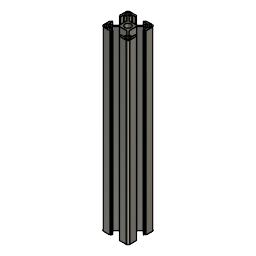
20cm profile beam (Autodesk Fusion 360 design; units mm, degrees)
Autodesk Fusion 360 part; units mm, degrees
sketch "Sketch1" plane through (0, 0, 0) normal (0, 0, 1) x (1, 0, 0)
  line L0 (-150, 300) -> (-150, 150) construction
  line L1 (0, 150) -> (-300, 150) construction
  line L2 (-205, 150) -> (-205, 192.65)
  line L3 (-191.8942, 205) -> (-108.1058, 205)
  line L4 (-95, 192.65) -> (-95, 150)
  line L5 (-150, 150) -> (-205, 205) construction
  line L6 (-150, 150) -> (-95, 205) construction
  line L7 (-205, 150) -> (-205, 192.65) construction
  line L8 (-280, 300) -> (-232.5, 300)
  line L9 (-232.5, 277) -> (-232.5, 246.4343)
  line L10 (-300, 232.5) -> (-300, 280)
  line L11 (-205, 192.65) -> (-244.2642, 231.9142)
  line L12 (-231.9142, 245.0201) -> (-191.8942, 205)
  line L13 (-279, 193) -> (-279, 232.5)
  line L14 (-288, 278) -> (-288, 150) construction
  line L15 (-278, 288) -> (-254.5, 288)
  line L16 (-244.5, 278) -> (-244.5, 254.5)
  line L17 (-254.5, 244.5) -> (-278, 244.5)
  arc A0 (-278, 288) -> (-288, 278) centre (-278, 278) ccw
  arc A1 (-244.5, 278) -> (-254.5, 288) centre (-254.5, 278) ccw
  arc A2 (-254.5, 244.5) -> (-244.5, 254.5) centre (-254.5, 254.5) ccw
  arc A3 (-288, 254.5) -> (-278, 244.5) centre (-278, 254.5) ccw
  line L18 (-288, 278) -> (-288, 254.5)
  line L19 (-191, 281) -> (-191, 286)
  line L20 (-200.9796, 290) -> (-200.9796, 298)
  line L21 (-193, 288) -> (-198.9796, 288)
  line L22 (-280, 300) -> (-202.9796, 300)
  line L23 (-230.5, 279) -> (-193, 279)
  line L24 (-279, 230.5) -> (-279, 191)
  line L25 (-288, 193) -> (-288, 198.6085)
  line L26 (-290, 200.6085) -> (-298, 200.6085)
  line L27 (-281, 191) -> (-286, 191)
  line L28 (-300, 280) -> (-300, 202.6085)
  line L29 (-288, 191) -> (-288, 288) construction
  line L30 (-245.6784, 232.5) -> (-277, 232.5)
  line L31 (-294.1421, 294.1421) -> (-285.0711, 285.0711) construction
  line L32 (-288, 288) -> (-285.0711, 285.0711) construction
  line L33 (-247.4289, 247.4289) -> (-150, 150) construction
  arc A4 (-200.9796, 298) -> (-202.9796, 300) centre (-202.9796, 298) ccw
  arc A5 (-191, 286) -> (-193, 288) centre (-193, 286) ccw
  arc A6 (-193, 279) -> (-191, 281) centre (-193, 281) ccw
  arc A7 (-200.9796, 290) -> (-198.9796, 288) centre (-198.9796, 290) ccw
  arc A8 (-230.5, 279) -> (-232.5, 277) centre (-230.5, 277) ccw
  arc A9 (-232.5, 246.4343) -> (-231.9142, 245.0201) centre (-230.5, 246.4343) ccw
  arc A10 (-244.2642, 231.9142) -> (-245.6784, 232.5) centre (-245.6784, 230.5) ccw
  line L34 (-300, 202.6085) -> (-300, 280)
  arc A11 (-288, 198.6085) -> (-290, 200.6085) centre (-290, 198.6085) ccw
  arc A12 (-288, 193) -> (-286, 191) centre (-286, 193) ccw
  arc A13 (-281, 191) -> (-279, 193) centre (-281, 193) ccw
  arc A14 (-277, 232.5) -> (-279, 230.5) centre (-277, 230.5) ccw
  arc A15 (-300, 202.6085) -> (-298, 200.6085) centre (-298, 202.6085) ccw
  arc A16 (-280, 300) -> (-300, 280) centre (-280, 280) ccw
  line L35 (-21, 193) -> (-21, 232.5)
  line L36 (-21, 230.5) -> (-21, 191)
  line L37 (-12, 191) -> (-12, 288) construction
  arc A17 (-12, 278) -> (-22, 288) centre (-22, 278) ccw
  line L38 (-68.0858, 245.0201) -> (-108.1058, 205)
  line L39 (0, 202.6085) -> (0, 280)
  arc A18 (-22, 244.5) -> (-12, 254.5) centre (-22, 254.5) ccw
  line L40 (-20, 300) -> (-97.0204, 300)
  line L41 (-95, 192.65) -> (-55.7358, 231.9142)
  arc A19 (0, 280) -> (-20, 300) centre (-20, 280) ccw
  line L42 (-107, 288) -> (-101.0204, 288)
  line L43 (-5.8579, 294.1421) -> (-14.9289, 285.0711) construction
  line L44 (-69.5, 279) -> (-107, 279)
  line L45 (-55.5, 278) -> (-55.5, 254.5)
  arc A20 (-68.0858, 245.0201) -> (-67.5, 246.4343) centre (-69.5, 246.4343) ccw
  line L46 (-20, 300) -> (-67.5, 300)
  line L47 (-54.3216, 232.5) -> (-23, 232.5)
  arc A21 (-55.5, 254.5) -> (-45.5, 244.5) centre (-45.5, 254.5) ccw
  arc A22 (-101.0204, 288) -> (-99.0204, 290) centre (-101.0204, 290) ccw
  line L48 (-67.5, 277) -> (-67.5, 246.4343)
  line L49 (-99.0204, 290) -> (-99.0204, 298)
  line L50 (0, 280) -> (0, 202.6085)
  arc A23 (-67.5, 277) -> (-69.5, 279) centre (-69.5, 277) ccw
  arc A24 (-45.5, 288) -> (-55.5, 278) centre (-45.5, 278) ccw
  arc A25 (-97.0204, 300) -> (-99.0204, 298) centre (-97.0204, 298) ccw
  arc A26 (-54.3216, 232.5) -> (-55.7358, 231.9142) centre (-54.3216, 230.5) ccw
  line L51 (-52.5711, 247.4289) -> (-150, 150) construction
  line L52 (-45.5, 244.5) -> (-22, 244.5)
  line L53 (-12, 288) -> (-14.9289, 285.0711) construction
  line L54 (0, 232.5) -> (0, 280)
  arc A27 (-21, 230.5) -> (-23, 232.5) centre (-23, 230.5) ccw
  line L55 (-22, 288) -> (-45.5, 288)
  line L56 (-12, 278) -> (-12, 254.5)
  arc A28 (-107, 288) -> (-109, 286) centre (-107, 286) ccw
  line L57 (-109, 281) -> (-109, 286)
  arc A29 (-109, 281) -> (-107, 279) centre (-107, 281) ccw
  line L58 (-10, 200.6085) -> (-2, 200.6085)
  arc A30 (-2, 200.6085) -> (0, 202.6085) centre (-2, 202.6085) ccw
  arc A31 (-10, 200.6085) -> (-12, 198.6085) centre (-10, 198.6085) ccw
  arc A32 (-14, 191) -> (-12, 193) centre (-14, 193) ccw
  line L59 (-19, 191) -> (-14, 191)
  arc A33 (-21, 193) -> (-19, 191) centre (-19, 193) ccw
  line L60 (-150, 150) -> (-247.4289, 247.4289) construction
  line L61 (-247.4289, 247.4289) -> (-150, 150) construction
  line L62 (0, 300) -> (-150, 150) construction
  line L63 (-12, 288) -> (-150, 150) construction
  line L64 (-150, 150) -> (-21, 279) construction
  line L65 (-150, 150) -> (-52.5711, 247.4289) construction
  line L66 (-52.5711, 247.4289) -> (-150, 150) construction
  arc A34 (-116, 150) -> (-184, 150) centre (-150, 150) ccw
  line L67 (-278, 12) -> (-254.5, 12)
  line L68 (-254.5, 55.5) -> (-278, 55.5)
  line L69 (-288, 22) -> (-288, 45.5)
  line L70 (-191, 19) -> (-191, 14)
  arc A35 (-245.6784, 67.5) -> (-244.2642, 68.0858) centre (-245.6784, 69.5) ccw
  line L71 (-279, 107) -> (-279, 67.5)
  arc A36 (-193, 12) -> (-191, 14) centre (-193, 14) ccw
  line L72 (-99.0204, 10) -> (-99.0204, 2)
  line L73 (-294.1421, 5.8579) -> (-285.0711, 14.9289) construction
  line L74 (-288, 107) -> (-288, 101.3915)
  line L75 (-300, 97.3915) -> (-300, 20)
  line L76 (-20, 0) -> (-97.0204, 0)
  arc A37 (-278, 55.5) -> (-288, 45.5) centre (-278, 45.5) ccw
  line L77 (-109, 19) -> (-109, 14)
  arc A38 (-232.5, 23) -> (-230.5, 21) centre (-230.5, 23) ccw
  line L78 (-193, 12) -> (-198.9796, 12)
  arc A39 (-254.5, 12) -> (-244.5, 22) centre (-254.5, 22) ccw
  arc A40 (-184, 150) -> (-116, 150) centre (-150, 150) ccw
  line L79 (-288, 12) -> (-285.0711, 14.9289) construction
  line L80 (-69.5, 21) -> (-107, 21)
  arc A41 (-300, 20) -> (-280, 0) centre (-280, 20) ccw
  line L81 (-290, 99.3915) -> (-298, 99.3915)
  arc A42 (-298, 99.3915) -> (-300, 97.3915) centre (-298, 97.3915) ccw
  arc A43 (-244.5, 45.5) -> (-254.5, 55.5) centre (-254.5, 45.5) ccw
  line L82 (-95, 107.35) -> (-55.7358, 68.0858)
  line L83 (-232.5, 23) -> (-232.5, 53.5657)
  line L84 (-245.6784, 67.5) -> (-277, 67.5)
  arc A44 (-99.0204, 2) -> (-97.0204, 0) centre (-97.0204, 2) ccw
  arc A45 (-288, 22) -> (-278, 12) centre (-278, 22) ccw
  arc A46 (-198.9796, 12) -> (-200.9796, 10) centre (-198.9796, 10) ccw
  line L85 (-288, 22) -> (-288, 150) construction
  line L86 (-300, 20) -> (-300, 97.3915)
  line L87 (-288, 109) -> (-288, 12) construction
  line L88 (-191.8942, 95) -> (-108.1058, 95)
  line L89 (-12, 22) -> (-12, 150) construction
  line L90 (-68.0858, 54.9799) -> (-108.1058, 95)
  arc A47 (-279, 107) -> (-281, 109) centre (-281, 107) ccw
  line L91 (-12, 150) -> (-12, 12) construction
  line L92 (-244.5, 22) -> (-244.5, 45.5)
  arc A48 (-290, 99.3915) -> (-288, 101.3915) centre (-290, 101.3915) ccw
  line L93 (-150, 0) -> (-150, 150) construction
  arc A49 (-107, 21) -> (-109, 19) centre (-107, 19) ccw
  arc A50 (-109, 14) -> (-107, 12) centre (-107, 14) ccw
  line L94 (-52.5711, 52.5711) -> (-150, 150) construction
  line L95 (0, 0) -> (-150, 150) construction
  line L96 (-150, 150) -> (-52.5711, 52.5711) construction
  line L97 (-150, 150) -> (-95, 95) construction
  line L98 (-107, 12) -> (-101.0204, 12)
  line L99 (-281, 109) -> (-286, 109)
  line L100 (-247.4289, 52.5711) -> (-150, 150) construction
  line L101 (-45.5, 55.5) -> (-22, 55.5)
  line L102 (-200.9796, 10) -> (-200.9796, 2)
  line L103 (-300, 67.5) -> (-300, 20)
  arc A51 (-69.5, 21) -> (-67.5, 23) centre (-69.5, 23) ccw
  arc A52 (-286, 109) -> (-288, 107) centre (-286, 107) ccw
  line L104 (-67.5, 23) -> (-67.5, 53.5657)
  line L105 (-231.9142, 54.9799) -> (-191.8942, 95)
  line L106 (-230.5, 21) -> (-193, 21)
  line L107 (-205, 150) -> (-205, 107.35)
  line L108 (0, 97.3915) -> (0, 20)
  line L109 (-247.4289, 52.5711) -> (-150, 150) construction
  line L110 (-205, 107.35) -> (-244.2642, 68.0858)
  line L111 (-279, 69.5) -> (-279, 109)
  arc A53 (-22, 12) -> (-12, 22) centre (-22, 22) ccw
  arc A54 (-191, 19) -> (-193, 21) centre (-193, 19) ccw
  arc A55 (-99.0204, 10) -> (-101.0204, 12) centre (-101.0204, 10) ccw
  line L112 (-205, 150) -> (-205, 107.35) construction
  line L113 (-12, 12) -> (-150, 150) construction
  line L114 (-52.5711, 52.5711) -> (-150, 150) construction
  arc A56 (-202.9796, 0) -> (-200.9796, 2) centre (-202.9796, 2) ccw
  arc A57 (-279, 69.5) -> (-277, 67.5) centre (-277, 69.5) ccw
  line L115 (-280, 0) -> (-202.9796, 0)
  line L116 (-150, 150) -> (-21, 21) construction
  line L117 (-280, 0) -> (-232.5, 0)
  line L118 (-95, 107.35) -> (-95, 150)
  arc A58 (-231.9142, 54.9799) -> (-232.5, 53.5657) centre (-230.5, 53.5657) ccw
  line L119 (-5.8579, 5.8579) -> (-14.9289, 14.9289) construction
  arc A59 (-12, 107) -> (-14, 109) centre (-14, 107) ccw
  arc A60 (-12, 101.3915) -> (-10, 99.3915) centre (-10, 101.3915) ccw
  arc A61 (-67.5, 53.5657) -> (-68.0858, 54.9799) centre (-69.5, 53.5657) ccw
  line L120 (0, 67.5) -> (0, 20)
  line L121 (-10, 99.3915) -> (-2, 99.3915)
  line L122 (0, 20) -> (0, 97.3915)
  line L123 (-150, 150) -> (-247.4289, 52.5711) construction
  arc A62 (-55.5, 22) -> (-45.5, 12) centre (-45.5, 22) ccw
  line L124 (-22, 12) -> (-45.5, 12)
  line L125 (-12, 22) -> (-12, 45.5)
  line L126 (-20, 0) -> (-67.5, 0)
  line L127 (-12, 109) -> (-12, 12) construction
  line L128 (-21, 69.5) -> (-21, 109)
  arc A63 (-55.7358, 68.0858) -> (-54.3216, 67.5) centre (-54.3216, 69.5) ccw
  line L129 (-19, 109) -> (-14, 109)
  arc A64 (-20, 0) -> (0, 20) centre (-20, 20) ccw
  line L130 (-54.3216, 67.5) -> (-23, 67.5)
  arc A65 (0, 97.3915) -> (-2, 99.3915) centre (-2, 97.3915) ccw
  arc A66 (-23, 67.5) -> (-21, 69.5) centre (-23, 69.5) ccw
  arc A67 (-45.5, 55.5) -> (-55.5, 45.5) centre (-45.5, 45.5) ccw
  line L131 (-21, 107) -> (-21, 67.5)
  arc A68 (-12, 45.5) -> (-22, 55.5) centre (-22, 45.5) ccw
  line L132 (-12, 12) -> (-14.9289, 14.9289) construction
  line L133 (-150, 150) -> (-205, 95) construction
  line L134 (-55.5, 22) -> (-55.5, 45.5)
  arc A69 (-19, 109) -> (-21, 107) centre (-19, 107) ccw
  line L135 (-12, 198.6085) -> (-12, 193)
  line L136 (-12, 107) -> (-12, 101.3915)
  point P0 (-150, 150)
  point P1 (-150, 150)
  point P2 (-150, 150)
  point P3 (-150, 150)
  point P4 (-150, 150)
  point P5 (-150, 150)
  point P6 (-300, 150)
  point P7 (0, 150)
  dimension "d1" = 300
  dimension "d5" = 42.65
  dimension "d10" = 18
  dimension "d11" = 21
  dimension "d13" = 12
  dimension "d15" = 10
  dimension "d16" = 10
  dimension "d17" = 10
  dimension "d19" = 2
  dimension "d20" = 2
  dimension "d21" = 2
  dimension "d22" = 2
  dimension "d23" = 2
  dimension "d24" = 2
  dimension "d25" = 2
  dimension "d26" = 2
  dimension "d27" = 2
  dimension "d28" = 2
  dimension "d29" = 2
  dimension "d30" = 20
  constraint horizontal L22
  constraint midpoint L1 P4
  constraint parallel L2 L4
  constraint coincident L5 P5
  constraint coincident L6 P5
  constraint coincident P4 P3
  constraint perpendicular L1 L7
  constraint horizontal L8
  constraint vertical L9
  constraint horizontal L30
  constraint vertical L10
  constraint parallel L11 L31
  constraint parallel L12 L31
  constraint coincident P5 P4
  constraint coincident P5 L63
  constraint coincident P5 L32
  constraint coincident L37.end L62
  constraint horizontal L15
  constraint vertical L16
  constraint horizontal L17
  constraint coincident L29.end L15
  constraint coincident L29.end L14
  constraint tangent L15 A0
  constraint tangent L14 A0
  constraint tangent L15 A1
  constraint tangent L16 A1
  constraint tangent L16 A2
  constraint tangent L17 A2
  constraint tangent L17 A3
  constraint tangent A3 L18
  constraint perpendicular L20 L22
  constraint coincident L0.start L22
  constraint symmetric L29.end L32.start L31
  constraint coincident A2 L33.start
  constraint coincident A0 L31.end
  constraint collinear L31 L61
  constraint collinear L32 L33
  constraint tangent L20 A4
  constraint tangent L22 A4
  constraint tangent L19 A5
  constraint tangent L21 A5
  constraint tangent L19 A6
  constraint tangent L23 A6
  constraint tangent L20 A7
  constraint tangent L21 A7
  constraint equal A6 A7
  constraint tangent L9 A8
  constraint tangent L23 A8
  constraint tangent L12 A9
  constraint tangent L9 A9
  constraint tangent L11 A10
  constraint tangent L30 A10
  constraint tangent L25 A11
  constraint tangent L26 A11
  constraint coincident L29.start L27
  constraint coincident L29.start L25
  constraint tangent L27 A12
  constraint tangent L25 A12
  constraint coincident L24.end L27
  constraint tangent L13 A13
  constraint tangent L27 A13
  constraint coincident L13.end L30
  constraint coincident L24 L13.end
  constraint tangent L30 A14
  constraint tangent L24 A14
  constraint tangent L28 A15
  constraint tangent L26 A15
  constraint tangent L22 A16
  constraint tangent L34 A16
  constraint coincident A16 L31.start
  constraint symmetric L0 L2.end L4.start
  constraint symmetric L0 L8.end L46.end
  constraint symmetric L0 L10.start L54.start
  constraint symmetric L0 L3.start L3.end
  constraint symmetric L0 L29.end L37.end
  constraint symmetric L0 L15.start A17.end
  constraint symmetric L0 L14.start A17.start
  constraint symmetric L0 A0 A17
  constraint symmetric L0 L15.end A24.start
  constraint symmetric L0 L16.start L45.start
  constraint symmetric L0 A1 A24
  constraint symmetric L0 L16.end L45.end
  constraint symmetric L0 L17.start A21.end
  constraint symmetric L0 A2 A21
  constraint symmetric L0 L17.end A18.start
  constraint symmetric L0 A3.start A18.end
  constraint symmetric L0 A3 A18
  constraint symmetric L0 L29.start L37.start
  constraint symmetric L0 L24.end L36.end
  constraint symmetric L0 L13.end L35.end
  constraint symmetric L0 L33.start L51.start
  constraint symmetric L0 L31.end L43.end
  constraint symmetric L0 L20.end L49.end
  constraint symmetric L0 L22.end L40.end
  constraint symmetric L0 A4 A25
  constraint symmetric L0 L19.end A28.end
  constraint symmetric L0 L21.start L42.start
  constraint symmetric L0 A5 A28
  constraint symmetric L0 L19.start L57.start
  constraint symmetric L0 L23.end L44.end
  constraint symmetric L0 A6 A29
  constraint symmetric L0 L20.start A22.end
  constraint symmetric L0 L21.end L42.end
  constraint symmetric L0 A7 A22
  constraint symmetric L0 L9.start L48.start
  constraint symmetric L0 L23.start L44.start
  constraint symmetric L0 A8 A23
  constraint symmetric L0 L12.start L38.start
  constraint symmetric L0 L9.end A20.end
  constraint symmetric L0 A9 A20
  constraint symmetric L0 L11.end L41.end
  constraint symmetric L0 L30.start L47.start
  constraint symmetric L0 A10 A26
  constraint symmetric L0 L25.end A31.end
  constraint symmetric L0 L26.start L58.start
  constraint symmetric L0 A11 A31
  constraint symmetric L0 L27.end A32.start
  constraint symmetric L0 L25.start A32.end
  constraint symmetric L0 A12 A32
  constraint symmetric L0 L13.start L35.start
  constraint symmetric L0 L27.start L59.start
  constraint symmetric L0 A13 A33
  constraint symmetric L0 L30.end L47.end
  constraint symmetric L0 L24.start L36.start
  constraint symmetric L0 A14 A27
  constraint symmetric L0 L28.end L39.start
  constraint symmetric L0 L26.end L58.end
  constraint symmetric L0 A15 A30
  constraint symmetric L0 L8.start L40.start
  constraint symmetric L0 L10.end L39.end
  constraint symmetric L0 A16 A19
  constraint symmetric L0 L31.start L43.start
  constraint coincident L1 L4.end
  constraint coincident L1 A34.end
  constraint coincident L1 A34.start
  constraint coincident L1 L14.end
  constraint symmetric L62.start L1 L95.start
  constraint symmetric L0.start L1 L93.start
  constraint symmetric P7 L1 L1.start
  constraint symmetric P6 L1 L1.end
  constraint symmetric L1 P4 P3
  constraint symmetric L1 L5.end L133.end
  constraint symmetric L1 L6.end L97.end
  constraint symmetric L1 P5 P4
  constraint symmetric L1 L2.start L7.start
  constraint symmetric L1 L2.end L107.end
  constraint symmetric L1 L8.end L117.end
  constraint symmetric L1 L10.start L103.start
  constraint symmetric L1 L3.start L88.start
  constraint symmetric L1 L64.end L116.end
  constraint symmetric L1 L37.end L91.end
  constraint symmetric L1 L29.end L79.start
  constraint symmetric L1 L15.start L67.start
  constraint symmetric L1 L14.start L69.start
  constraint symmetric L1 A0 A45
  constraint symmetric L1 L15.end L67.end
  constraint symmetric L1 L16.start A39.end
  constraint symmetric L1 A1 A39
  constraint symmetric L1 L16.end A43.start
  constraint symmetric L1 L17.start L68.start
  constraint symmetric L1 A2 A43
  constraint symmetric L1 L17.end L68.end
  constraint symmetric L1 A3.start L69.end
  constraint symmetric L1 A3 A37
  constraint symmetric L1 L29.start L87.start
  constraint symmetric L1 L24.end L111.end
  constraint symmetric L1 L13.end L71.end
  constraint symmetric L1 L33.start L100.start
  constraint symmetric L1 L31.end L73.end
  constraint symmetric L1 L20.end L102.end
  constraint symmetric L1 L22.end A56.start
  constraint symmetric L1 A4 A56
  constraint symmetric L1 L19.end L70.end
  constraint symmetric L1 L21.start A36.start
  constraint symmetric L1 A5 A36
  constraint symmetric L1 L19.start L70.start
  constraint symmetric L1 L23.end L106.end
  constraint symmetric L1 A6 A54
  constraint symmetric L1 L20.start A46.end
  constraint symmetric L1 L21.end L78.end
  constraint symmetric L1 A7 A46
  constraint symmetric L1 L9.start A38.start
  constraint symmetric L1 L23.start A38.end
  constraint symmetric L1 A8 A38
  constraint symmetric L1 L12.start L105.start
  constraint symmetric L1 L9.end L83.end
  constraint symmetric L1 A9 A58
  constraint symmetric L1 L11.end A35.end
  constraint symmetric L1 L30.start A35.start
  constraint symmetric L1 A10 A35
  constraint symmetric L1 L25.end L74.end
  constraint symmetric L1 L26.start L81.start
  constraint symmetric L1 A11 A48
  constraint symmetric L1 L27.end L99.end
  constraint symmetric L1 L25.start L74.start
  constraint symmetric L1 A12 A52
  constraint symmetric L1 L13.start L71.start
  constraint symmetric L1 L27.start A47.end
  constraint symmetric L1 A13 A47
  constraint symmetric L1 L30.end L84.end
  constraint symmetric L1 L24.start L111.start
  constraint symmetric L1 A14 A57
  constraint symmetric L1 L28.end L75.start
  constraint symmetric L1 L26.end L81.end
  constraint symmetric L1 A15 A42
  constraint symmetric L1 L8.start A41.end
  constraint symmetric L1 L10.end L75.end
  constraint symmetric L1 A16 A41
  constraint symmetric L1 L31.start L73.start
  constraint symmetric L1 L43.start L119.start
  constraint symmetric L1 L47.start A63.end
  constraint symmetric L1 L39.end L108.end
  constraint symmetric L1 L43.end L119.end
  constraint symmetric L1 L35.end L131.end
  constraint symmetric L1 L40.start L76.start
  constraint symmetric L1 L47.end L130.end
  constraint symmetric L1 L54.start L120.start
  constraint symmetric L1 L36.start L128.start
  constraint symmetric L1 L49.end L72.end
  constraint symmetric L1 L40.end L76.end
  constraint symmetric L1 L45.end A67.end
  constraint symmetric L1 A21.end L101.start
  constraint symmetric L1 A22.end L72.start
  constraint symmetric L1 L42.end L98.end
  constraint symmetric L1 A17.start L89.start
  constraint symmetric L1 L48.start A51.end
  constraint symmetric L1 L45.start A62.start
  constraint symmetric L1 A17.end A53.start
  constraint symmetric L1 L38.start L90.start
  constraint symmetric L1 A24.start A62.end
  constraint symmetric L1 L44.start L80.start
  constraint symmetric L1 L41.end L82.end
  constraint symmetric L1 A18.start L101.end
  constraint symmetric L1 A18.end L125.end
  constraint symmetric L1 L51.start L94.start
  constraint symmetric L1 L46.end L126.end
  constraint symmetric L1 A20.end L104.end
  constraint symmetric L1 A28.end L77.end
  constraint symmetric L1 L35.start L131.start
  constraint symmetric L1 L36.end L128.end
  constraint symmetric L1 L37.start L127.start
  constraint symmetric L1 A17 A53
  constraint symmetric L1 L3.end L88.end
  constraint symmetric L1 A18 A68
  constraint symmetric L1 L4.start L82.start
  constraint symmetric L1 A19 A64
  constraint symmetric L1 L42.start A50.end
  constraint symmetric L1 L44.end L80.end
  constraint symmetric L1 A20 A61
  constraint symmetric L1 A21 A67
  constraint symmetric L1 A22 A55
  constraint symmetric L1 L39.start L108.start
  constraint symmetric L1 A23 A51
  constraint symmetric L1 A24 A62
  constraint symmetric L1 A25 A44
  constraint symmetric L1 A26 A63
  constraint symmetric L1 A27 A66
  constraint symmetric L1 A28 A50
  constraint symmetric L1 L57.start L77.start
  constraint symmetric L1 A29 A49
  constraint symmetric L1 L58.start A60.end
  constraint symmetric L1 L58.end L121.end
  constraint symmetric L1 A30 A65
  constraint symmetric L1 A31.end A60.start
  constraint symmetric L1 A31 A60
  constraint symmetric L1 A32.end A59.start
  constraint symmetric L1 A32.start A59.end
  constraint symmetric L1 A32 A59
  constraint symmetric L1 L59.start L129.start
  constraint symmetric L1 A33 A69
  constraint symmetric L1 L4.end L118.end
  constraint symmetric L1 A34.end A40.start
  constraint symmetric L1 A34 A40
  constraint symmetric L1 A34.start A40.end
  constraint symmetric L1 L14.end L85.end
  measures "d1" distance of L95.start L62.start
  measures "d5" distance of L2.start L2.end
  measures "d10" distance of L11 L12
  measures "d11" distance of L22 L23
  measures "d13" distance of L9 L16
  measures "d15" radius of A1
  measures "d16" radius of A2
  measures "d17" radius of A3
  measures "d19" radius of A4
  measures "d20" radius of A5
  measures "d21" radius of A6
  measures "d22" radius of A8
  measures "d23" radius of A9
  measures "d24" radius of A10
  measures "d25" radius of A11
  measures "d26" radius of A12
  measures "d27" radius of A13
  measures "d28" radius of A14
  measures "d29" radius of A15
  measures "d30" radius of A16
extrude "Extrude1" add sketch "Sketch1" along normal blind 2000
scale "Scale1" factor 0.1 about (-108.1058, 95, 0) bodies 1
scale "Scale2" factor 0.666667 about (-108.1058, 95, 0) bodies 1
equation "d5 = ( 85.3 / 2 ) * 1 mm"
equation "d34 = 1 / 1.5"
